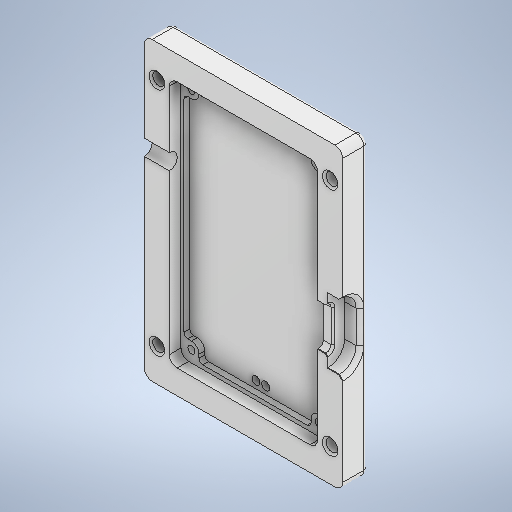
# Autodesk Inventor part: universal_case_back
Saved by Autodesk Inventor 2025 (Build 290162010, 162A)
## iProperties
Created: 2025-11-15
Part Number: universal_case_back
Material: PC/ABS Plastic
Document SubType Name: Modeling
Designer: vaugerbird
Density: 1.1 g/cm^3
Appearance: Smooth - White
Author: vaugerbird
Autodesk Inventor part; units mm, degrees
ref_plane "YZ Plane" through (0, 0, 0) normal (1, 0, 0) x (0, 1, 0)
ref_plane "XZ Plane" through (0, 0, 0) normal (0, 1, 0) x (-1, 0, 0)
ref_plane "XY Plane" through (0, 0, 0) normal (0, 0, 1) x (1, 0, 0)
sketch "Sketch1" plane through (0, 0, 0) normal (0, 0, 1) x (1, 0, 0)
  line L0 (9.24, 67.66) -> (9.24, 9.24)
  line L1 (42.26, 9.239739) -> (42.26, 67.66)
  line L2 (51.5, 2) -> (51.5, 74.9)
  line L3 (47.5, 28.739684) -> (45, 28.739684)
  line L4 (51.5, 30.039684) -> (51.5, 9.574945)
  line L5 (9.24, 9.24) -> (42.26, 9.239739)
  line L6 (47.5, 28.239684) -> (47.5, 28.739684)
  line L7 (47.5, 25.739684) -> (47.5, 28.239684)
  line L8 (47.5, 25.739684) -> (51.5, 25.739684)
  line L9 (47.5, 39.739684) -> (47, 39.739684)
  line L10 (45, 39.739684) -> (47, 39.739684)
  circle A0 centre (9.24, 9.24) radius 0.95
  circle A1 centre (42.26, 9.239739) radius 0.95
  line L11 (51.5, 38.439684) -> (51.5, 43.739684)
  line L12 (47.5, 42.739684) -> (47.5, 39.739684)
  line L13 (6.5, 53.709945) -> (6.5, 49.609945)
  line L14 (6.5, 49.609945) -> (0, 49.609945)
  line L15 (0, 49.609945) -> (6.5, 49.609945)
  line L16 (0, 53.709945) -> (6.5, 53.709945)
  line L17 (45, 39.739684) -> (47.5, 39.739684)
  line L18 (47.5, 42.739684) -> (51.5, 42.739684)
  line L19 (42.26, 67.66) -> (9.24, 67.66)
  circle A2 centre (9.24, 67.66) radius 0.95
  circle A3 centre (42.26, 67.66) radius 0.95
  line L20 (6.5, 53.709945) -> (6.5, 49.609945)
  line L21 (6.5, 68.4) -> (6.5, 8.5)
  circle A4 centre (48.25, 68.4) radius 1.55
  circle A5 centre (3.25, 68.4) radius 1.55
  line L22 (25.75, 70.4) -> (25.75, 76.9)
  line L23 (25.75, 76.9) -> (49.5, 76.9)
  line L24 (25.75, 76.9) -> (2, 76.9)
  arc A6 (2, 76.9) -> (0, 74.9) centre (2, 74.9) ccw
  arc A7 (51.5, 74.9) -> (49.5, 76.9) centre (49.5, 74.9) ccw
  line L25 (45, 8.25) -> (45, 68.40013)
  line L26 (25.75, 6.5) -> (25.75, 0)
  line L27 (25.75, 0) -> (49.5, 0)
  line L28 (25.75, 0) -> (2, 0)
  arc A8 (0, 1.99987) -> (2, 0) centre (2, 2) ccw
  arc A9 (49.5, 0) -> (51.5, 2) centre (49.5, 2) ccw
  line L29 (3.25, 0) -> (3.25, 8.5)
  line L30 (48.25, 0) -> (48.25, 8.5)
  circle A10 centre (48.25, 8.5) radius 1.55
  circle A11 centre (3.25, 8.5) radius 1.55
  line L31 (0, 1.99987) -> (0, 0)
  line L32 (0, 1.99987) -> (0, 74.9)
  line L33 (25.75, 6.5) -> (25.75, 70.4)
  line L34 (2, 0) -> (0, 0)
  line L35 (9.24, 9.24) -> (6.5, 9.24)
  line L36 (6.5, 9.24) -> (6.5, 8.99)
  line L37 (6.5, 8.99) -> (6.5, 8.25)
  line L38 (8.5, 6.25) -> (43, 6.25)
  line L39 (45, 6.25) -> (45, 8.5)
  arc A12 (6.5, 8.25) -> (8.5, 6.25) centre (8.5, 8.25) ccw
  arc A13 (43, 6.25) -> (45, 8.25) centre (43, 8.25) ccw
  line L40 (9.24, 67.66) -> (6.5, 67.66)
  line L41 (6.5, 67.66) -> (6.5, 67.91)
  line L42 (6.5, 67.91) -> (6.5, 68.65)
  line L43 (8.5, 70.65) -> (43, 70.65)
  line L44 (45, 68.65) -> (45, 67.66)
  arc A14 (8.5, 70.65) -> (6.5, 68.65) centre (8.5, 68.65) ccw
  arc A15 (45, 68.65) -> (43, 70.65) centre (43, 68.65) ccw
  point P0 (6.5, 70.4)
  point P1 (0, 76.9)
  point P2 (6.5, 6.5)
  point P3 (6.5, 6.25)
  point P4 (6.5, 70.65)
  dimension "d21" = 6.5
  dimension "d24" = 3.1
  dimension "d25" = 3.1
  dimension "d27" = 2
  dimension "d31" = 2
  dimension "d32" = 8.5
  dimension "d33" = 8.5
  dimension "d34" = 3.1
  dimension "d35" = 3.1
  dimension "d36" = 72.90013
  dimension "d110" = 1.99987
  dimension "d111" = 23.75
  dimension "d113" = 0.25
  dimension "d114" = 2.74
  dimension "d115" = 2
  dimension "d116" = 0.25
  dimension "d117" = 2.74
  dimension "d118" = 2
  constraints: 90 end point, 23 point on line, 17 point on circle, 16 centre point, 16 tangent, 8 perpendicular, 7 vertical, 4 collinear, 4 equal radius, 2 coincident, 1 horizontal, 1 parallel
  measures "d21" distance of L16.start L13.start
  measures "d24" diameter of A4
  measures "d25" diameter of A5
  measures "d27" radius of A6
  measures "d31" radius of A8
  measures "d32" distance of L29.start L29.end
  measures "d33" distance of L30.start L30.end
  measures "d34" diameter of A10
  measures "d35" diameter of A11
  measures "d36" distance of L31.start L32.end
  measures "d110" distance of L31.start L31.end
  measures "d111" distance of L26.end L28.end
  measures "d113" distance of L35.end L36.end
  measures "d114" distance of L36.end point (6.5, 6.25)
  measures "d115" radius of A12
  measures "d116" distance of L40.end L41.end
  measures "d117" distance of L41.end point (6.5, 70.65)
  measures "d118" radius of A14
extrude "Extrusion1" add sketch "Sketch1" against normal blind 6.5 contours L19 A2 L0 | L40 A2 L19 | L0 A2 L40 | A2 L19 L33 L5 A0 L0 | L0 A0 L35 L21 L13 L40 A2 | A2 L40 L21 L42 A14 L43 L22 L33 L19 | A0 L5 L0 | L0 L35 A0 | L33 L22 L43 A15 L44 L25 A13 L38 L26 L5 A1 L1 A3 L19 | L19 A3 L1 A1 L5 L33 | L21 L16 L32 A6 L24 L22 L43 A14 L42 | L5 A0 L35 | L5 L33 L26 L38 A12 L37 L21 L35 A0 | A3 L1 L19 | L19 L1 A3 | L13 L14 L32 L16 | L21 L37 A12 L38 L26 L28 A8 L32 L14 | A1 L1 L5 | L5 L1 A1 | L22 L23 A7 L2 L18 L12 L9 L10 L25 L44 A15 L43 | L38 A13 L25 L3 L6 L7 L8 L2 A9 L27 L26 | L25 L10 L9 L12 L18 L2 L8 L7 L6 L3 | A4 | A5 | A10 | A11
extrude "Extrusion2" cut sketch "Sketch1" against normal blind 3 contours L19 A2 L0 | L40 A2 L19 | L0 A2 L40 | A2 L19 L33 L5 A0 L0 | L0 A0 L35 L21 L13 L40 A2 | A2 L40 L21 L42 A14 L43 L22 L33 L19 | A0 L5 L0 | L0 L35 A0 | L33 L22 L43 A15 L44 L25 A13 L38 L26 L5 A1 L1 A3 L19 | L19 A3 L1 A1 L5 L33 | L5 A0 L35 | L5 L33 L26 L38 A12 L37 L21 L35 A0 | A3 L1 L19 | L19 L1 A3 | A1 L1 L5 | L5 L1 A1
extrude "Extrusion3" cut sketch "Sketch1" against normal blind 4.5 contours A4 | A5 | A10 | A11
sketch "Sketch2" plane through (0, 0, -3) normal (0, 0, 1) x (1, 0, 0)
  line L0 (43, 6.5) -> (8.5, 6.5)
  line L1 (8.5, 6.5) -> (8.5, 9.24)
  line L2 (6.5, 8.25) -> (6.5, 68.65)
  line L3 (6.5, 8.5) -> (9.24, 8.5)
  line L4 (9.24, 8.5) -> (9.24, 9.24)
  line L5 (9.24, 9.24) -> (8.5, 9.24)
  circle A0 centre (9.24, 9.24) radius 0.95
  line L6 (9.24, 9.24) -> (25.75, 9.24)
  line L7 (8.5, 70.4) -> (43, 70.4)
  arc A1 (42.26, 11.19) -> (40.31, 9.24) centre (42.26, 9.24) ccw
  arc A2 (9.24, 65.71) -> (11.190033, 67.66) centre (9.240033, 67.66) ccw
  arc A3 (40.310033, 67.66) -> (42.260033, 65.71) centre (42.260033, 67.66) ccw
  line L8 (6.5, 11.19) -> (7.29, 11.19)
  line L9 (7.29, 12.19) -> (7.29, 64.71)
  line L10 (8.29, 65.71) -> (9.240067, 65.71)
  line L11 (11.190033, 70.4) -> (11.190033, 69.61)
  line L12 (11.190033, 68.61) -> (11.190033, 67.66)
  line L13 (12.190033, 69.61) -> (39.310033, 69.61)
  line L14 (40.310033, 68.61) -> (40.310033, 67.66)
  line L15 (45, 68.65) -> (45, 8.25)
  line L16 (45, 65.71) -> (44.21, 65.71)
  line L17 (45, 65.71) -> (45.79, 65.71) construction
  line L18 (43.21, 65.71) -> (42.260033, 65.71)
  line L19 (44.21, 64.71) -> (44.21, 12.19)
  line L20 (43.21, 11.19) -> (42.26, 11.19)
  line L21 (40.31, 6.5) -> (40.31, 7.29)
  line L22 (40.31, 8.29) -> (40.31, 9.24)
  line L23 (39.31, 7.29) -> (12.19, 7.29)
  line L24 (11.19, 8.29) -> (11.19, 9.24)
  line L25 (8.29, 11.19) -> (9.24, 11.19)
  arc A4 (11.19, 8.29) -> (12.19, 7.29) centre (12.19, 8.29) ccw
  arc A5 (7.29, 12.19) -> (8.29, 11.19) centre (8.29, 12.19) ccw
  arc A6 (39.31, 7.29) -> (40.31, 8.29) centre (39.31, 8.29) ccw
  arc A7 (43.21, 11.19) -> (44.21, 12.19) centre (43.21, 12.19) ccw
  arc A8 (44.21, 64.71) -> (43.21, 65.71) centre (43.21, 64.71) ccw
  arc A9 (40.310033, 68.61) -> (39.310033, 69.61) centre (39.310033, 68.61) ccw
  arc A10 (12.190033, 69.61) -> (11.190033, 68.61) centre (12.190033, 68.61) ccw
  arc A11 (8.29, 65.71) -> (7.29, 64.71) centre (8.29, 64.71) ccw
  arc A12 (7.435866, 8.5) -> (8.5, 7.435866) centre (9.24, 9.24) ccw
  arc A13 (11.19, 9.24) -> (9.24, 11.19) centre (9.24, 9.24) ccw
  point P0 (0, 0)
  point P1 (6.5, 68.4)
  point P2 (40.310033, 69.61)
  point P3 (45, 68.40013)
  point P4 (45, 8.5)
  dimension "d44" = 2.74
  dimension "d45" = 2.74
  dimension "d46" = 1.9
  dimension "d48" = 0.79
  dimension "d49" = 0.79
  dimension "d50" = 1.95
  dimension "d51" = 0.79
  dimension "d52" = 180
  dimension "d53" = 0.79
  dimension "d54" = 1
  constraints: 44 end point, 27 point on circle, 21 point on line, 19 tangent, 14 centre point, 7 equal radius, 6 perpendicular, 4 horizontal, 4 vertical, 2 coincident, 1 collinear, 1 parallel
  measures "d44" distance of L0.end L1.end
  measures "d45" distance of L3.start L3.end
  measures "d46" diameter of A0
  measures "d48" distance of L8.start L8.end
  measures "d49" distance of L11.start L11.end
  measures "d50" distance of point (40.31, 69.61) L14.end
  measures "d51" distance of L16.start L16.end
  measures "d52" angle of L16 L17
  measures "d53" distance of L21.start L21.end
  measures "d54" radius of A4
extrude "Extrusion4" cut sketch "Sketch2" against normal blind 1.5 contours A1 L22 A6 L23 A4 L24 A13 L25 A5 L9 A11 L10 A2 L12 A10 L13 A9 L14 A3 L18 A8 L19 A7 L20
extrude "Extrusion5" cut sketch "Sketch1" against normal up to surface (6.5 mm away) contours L19 A2 L0 | L40 A2 L19 | L0 A2 L40 | A0 L5 L0 | L0 L35 A0 | L5 A0 L35 | A3 L1 L19 | L19 L1 A3 | A1 L1 L5 | L5 L1 A1
sketch "Sketch3" plane through (0, 1.99987, 0) normal (-1, 0, 0) x (0, 0, 1)
  line L0 (0, 72.90013) -> (0, 74.90013)
  line L1 (0, 74.90013) -> (0, 51.71013)
  line L2 (0, 51.71013) -> (0, 47.61013)
  line L3 (0, 6.25013) -> (0, 66.65013)
  line L4 (0, 47.61013) -> (0, 49.66013)
  circle A0 centre (0, 49.66013) radius 2.05
  point P0 (0, -1.99987)
  point P1 (0, 6.50013)
  point P2 (0, 66.40013)
  dimension "d59" = 23.19
  dimension "d60" = 4.1
  constraints: 6 end point, 1 coincident, 1 midpoint, 1 point on line, 1 vertical, 3 other
  measures "d59" distance of L0.end L1.end
  measures "d60" distance of L1.end L2.end
extrude "Extrusion6" cut sketch "Sketch3" against normal up to surface (6.5 mm away) contours L2 A0 picked at (-0.163532, 48.31332)
sketch "Sketch4" plane through (51.5, 2, 0) normal (1, 0, 0) x (0, 0, -1)
  line L0 (0, 74.9) -> (0, 72.9) projected
  line L1 (0, 74.9) -> (0, 37.74)
  line L2 (0, 37.74) -> (0, 26.74)
  line L3 (0, 66.65) -> (0, 6.25) projected
  line L4 (0, 26.74) -> (0.2, 26.74)
  line L5 (1.5, 28.04) -> (1.5, 36.44)
  line L6 (0.2, 37.74) -> (0, 37.74)
  arc A0 (0.2, 26.74) -> (1.5, 28.04) centre (0.2, 28.04) ccw
  arc A1 (1.5, 36.44) -> (0.2, 37.74) centre (0.2, 36.44) ccw
  line L7 (4.5, 28.04) -> (4.5, 36.44)
  arc A2 (4.5, 36.44) -> (0.2, 40.74) centre (0.2, 36.44) ccw
  line L8 (0.2, 40.74) -> (0, 40.74)
  line L9 (0, 23.74) -> (0.2, 23.74)
  arc A3 (0.2, 23.74) -> (4.5, 28.04) centre (0.2, 28.04) ccw
  point P0 (0, -2)
  point P1 (0, 66.40013)
  point P2 (0, 6.5)
  point P3 (1.5, 26.74)
  dimension "d63" = 37.16
  dimension "d64" = 11
  dimension "d65" = 1.5
  dimension "d66" = 1.3
  dimension "d67" = 3
  constraints: 16 end point, 8 point on circle, 5 point on line, 4 centre point, 4 perpendicular, 4 tangent, 1 equal radius, 1 horizontal, 1 vertical, 1 other
  measures "d63" distance of L0.start L1.end
  measures "d64" distance of L1.end L2.end
  measures "d65" distance of L2.end point (1.5, 26.74)
  measures "d66" radius of A0
  measures "d67" radial gap between concentric circles of A0 A3
extrude "Extrusion7" cut sketch "Sketch4" against normal up to surface (6.5 mm away) contours L6 A1 L5 A0 L4 L2
extrude "Extrusion8" cut sketch "Sketch4" against normal blind 4 contours L8 A2 L7 A3 L9 L3 L4 A0 L5 A1 L6 L1
chamfer "Chamfer1" distance 1 angle 45 5 edges at (51.5, 34.24, -4.5) (51.5, 26.9994, -3.2406) (51.5, 25.74, -0.1) (51.5, 41.4806, -3.2406) (51.5, 42.74, -0.1)
chamfer "Chamfer2" distance 0.5 angle 45 9 edges at (47.5, 39.74, -0.1) (47.5, 39.3592, -1.1192) (47.5, 34.24, -1.5) (47.5, 29.1208, -1.1192) (47.5, 28.74, -0.1) (46.7, 68.4, 0) (46.7, 8.5, 0) (1.7, 8.5, 0) (1.7, 68.4, 0)
fillet "Fillet1" radius 1 8 edges at (51.5, 38.45, -6.5) (25.75, 0, -6.5) (50.9142, 0.5858, -6.5) (0, 38.4499, -6.5) (0.5858, 0.5857, -6.5) (25.75, 76.9, -6.5) (0.5858, 76.3142, -6.5) (50.9142, 76.3142, -6.5)
sketch "Sketch5" plane through (0, 0, -6.5) normal (0, 0, -1) x (-1, 0, 0)
  line L0 (-49.5, 75.9) -> (-2, 75.9)
  line L1 (-25.75, 75.9) -> (-25.75, 70.4)
  line L2 (-1, 74.9) -> (-1, 1.999935)
  line L3 (-25.75, 73.15) -> (-51.5, 73.15)
  line L4 (-51.5, 74.9) -> (-51.5, 38.44)
  line L5 (-51.5, 73.15) -> (-42.26, 73.15)
  circle A0 centre (-42.26, 73.15) radius 2.625
  line L6 (-25.75, 73.15) -> (0, 73.15)
  line L7 (0, 74.9) -> (0, 1.99987)
  arc A1 (0, 73.15) -> (0, 73.15) centre (0, 0) ccw
  line L8 (0, 73.15) -> (-9.24, 73.15)
  circle A2 centre (-9.24, 73.15) radius 2.625
  line L9 (-2, 1) -> (-49.5, 1)
  line L10 (-25.75, 1) -> (-25.75, 6.5)
  line L11 (-25.75, 3.75) -> (-51.5, 3.75)
  line L12 (-51.5, 2) -> (-51.5, 24.74)
  line L13 (-25.75, 3.75) -> (0, 3.75)
  line L14 (0, 74.9) -> (0, 1.99987)
  line L15 (-51.5, 3.75) -> (-42.26, 3.75)
  line L16 (0, 3.75) -> (-9.24, 3.75)
  circle A3 centre (-42.26, 3.75) radius 2.625
  circle A4 centre (-9.24, 3.75) radius 2.625
  point P0 (0, 0)
  point P1 (0, 53.71)
  point P2 (0, 49.61)
  dimension "d83" = 5.5
  dimension "d84" = 9.24
  dimension "d86" = 5.25
  dimension "d89" = 9.24
  dimension "d91" = 5.25
  dimension "d92" = 5.5
  dimension "d93" = 9.24
  dimension "d94" = 9.24
  dimension "d97" = 5.25
  dimension "d98" = 5.25
  constraints: 20 end point, 10 point on line, 5 centre point, 5 coincident, 4 midpoint, 3 horizontal, 2 point on circle, 2 vertical, 1 tangent
  measures "d83" distance of L1.start L1.end
  measures "d84" distance of L3.end L5.end
  measures "d86" diameter of A0
  measures "d89" distance of L8.start L8.end
  measures "d91" diameter of A2
  measures "d92" distance of L10.start L10.end
  measures "d93" distance of L11.end L15.end
  measures "d94" distance of L13.end L16.end
  measures "d97" diameter of A3
  measures "d98" diameter of A4
extrude "Extrusion9" cut sketch "Sketch5" against normal blind 2 contours A2 A1 L6 | L6 A2 | A2 A1 | A0 L3 | L3 A0 | A3 L11 | L11 A3 | L13 A4 | L13 A4
sketch "Sketch6" plane through (0, 0, -4.5) normal (0, 0, 1) x (1, 0, 0)
  circle A0 centre (42.26, 9.239739) radius 0.95
  line L0 (42.26, 9.239739) -> (27.025, 9.239739)
  circle A1 centre (9.24, 9.24) radius 0.95
  line L1 (9.24, 9.24) -> (24.48, 9.24)
  circle A2 centre (24.48, 9.24) radius 1.05
  circle A3 centre (27.025, 9.239739) radius 1.05
  circle A4 centre (24.48, 9.24) radius 1.2
  circle A5 centre (27.025, 9.239739) radius 1.2
  point P0 (0, 0)
  dimension "d102" = 15.235
  dimension "d103" = 15.24
  dimension "d104" = 2.1
  dimension "d105" = 2.1
  dimension "d106" = 2.4
  dimension "d107" = 2.4
  constraints: 4 centre point, 4 coincident, 4 end point, 2 horizontal
  measures "d102" distance of L0.start L0.end
  measures "d103" distance of L1.start L1.end
  measures "d104" diameter of A2
  measures "d105" diameter of A3
  measures "d106" diameter of A4
  measures "d107" diameter of A5
extrude "Extrusion10" cut sketch "Sketch6" against normal up to surface (2 mm away) contours A2 | A3
sketch "Sketch9" plane through (0, 0, -6.5) normal (0, 0, -1) x (-1, 0, 0)
  circle A0 centre (-42.26, 3.75) radius 2.625
  circle A1 centre (-9.24, 3.75) radius 2.625
  line L0 (-42.26, 3.75) -> (-9.24, 3.75)
  line L1 (-25.75, 3.75) -> (-16.125, 3.75)
  line L2 (-16.125, 3.75) -> (-16.125, 6)
  line L3 (-43, 6.25) -> (-8.5, 6.25)
  line L4 (-16.375, 6.25) -> (-35.125, 6.25)
  line L5 (-16.125, 3.75) -> (-16.125, 1.5)
  line L6 (-16.375, 1.25) -> (-35.125, 1.25)
  line L7 (-35.375, 1.5) -> (-35.375, 6)
  arc A2 (-35.125, 6.25) -> (-35.375, 6) centre (-35.125, 6) ccw
  arc A3 (-35.375, 1.5) -> (-35.125, 1.25) centre (-35.125, 1.5) ccw
  arc A4 (-16.375, 1.25) -> (-16.125, 1.5) centre (-16.375, 1.5) ccw
  arc A5 (-16.125, 6) -> (-16.375, 6.25) centre (-16.375, 6) ccw
  line L8 (-50.5, 2) -> (-50.5, 74.9)
  line L9 (-50.5, 38.45) -> (-1, 38.449967)
  line L10 (-1, 74.9) -> (-1, 1.999935)
  circle A6 centre (-42.259954, 73.149989) radius 2.625
  circle A7 centre (-9.239954, 73.149946) radius 2.625
  line L11 (-42.259954, 73.149989) -> (-9.239954, 73.149946)
  line L12 (-25.749954, 73.149967) -> (-16.124954, 73.149955)
  line L13 (-16.124954, 73.149955) -> (-16.124957, 70.899955)
  line L14 (-42.999958, 70.64999) -> (-8.499958, 70.649945)
  line L15 (-16.374958, 70.649955) -> (-35.124958, 70.64998)
  line L16 (-16.124954, 73.149955) -> (-16.124951, 75.399955)
  line L17 (-16.374951, 75.649955) -> (-35.124951, 75.64998)
  line L18 (-35.374951, 75.39998) -> (-35.374957, 70.89998)
  arc A8 (-35.374957, 70.89998) -> (-35.124958, 70.64998) centre (-35.124957, 70.89998) ccw
  arc A9 (-35.124951, 75.64998) -> (-35.374951, 75.39998) centre (-35.124951, 75.39998) ccw
  arc A10 (-16.124951, 75.399955) -> (-16.374951, 75.649955) centre (-16.374951, 75.399955) ccw
  arc A11 (-16.374958, 70.649955) -> (-16.124957, 70.899955) centre (-16.374957, 70.899955) ccw
  point P0 (0, 0)
  point P1 (-16.125, 6.25)
  point P2 (-35.375, 6.25)
  point P3 (-16.125, 1.25)
  point P4 (-16.124958, 70.649955)
  point P5 (-35.374958, 70.64998)
  point P6 (-16.124951, 75.649955)
  dimension "d122" = 9.625
  dimension "d123" = 2.5
  dimension "d124" = 19.25
  dimension "d125" = 2.5
  dimension "d126" = 0.25
  constraints: 32 end point, 21 symmetric about line, 16 point on circle, 14 point on line, 10 centre point, 8 tangent, 4 perpendicular, 3 equal radius, 3 midpoint, 1 horizontal, 1 vertical, 6 other
  measures "d122" distance of L1.start L1.end
  measures "d123" distance of L1.end point (-16.125, 6.25)
  measures "d124" distance of point (-16.125, 6.25) point (-35.375, 6.25)
  measures "d125" distance of L1.end point (-16.125, 1.25)
  measures "d126" radius of A2
extrude "Extrusion11" cut sketch "Sketch9" against normal blind 2 contours L7 A2 L3 A5 L2 L0 | L0 L5 A4 L6 A3 L7 | L18 A9 L17 A10 L16 L11 | L11 L13 A11 L14 A8 L18
fillet "Fillet2" radius 0.25 19 edges at (11.865, 3.75, -6.5) (44.885, 3.75, -6.5) (44.885, 73.15, -6.5) (11.865, 73.15, -6.5) (25.75, 6.25, -6.5) (35.3018, 6.1768, -6.5) (35.375, 3.75, -6.5) (35.3018, 1.3232, -6.5) (16.1982, 1.3232, -6.5) (16.125, 3.75, -6.5) (16.1982, 6.1768, -6.5) (35.375, 73.15, -6.5) (25.75, 75.65, -6.5) (25.75, 70.65, -6.5) (35.3017, 70.7232, -6.5) (35.3017, 75.5768, -6.5) (16.1982, 75.5767, -6.5) (16.125, 73.15, -6.5) (16.1982, 70.7232, -6.5)
body "Solid1"
